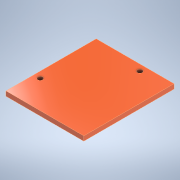
# Autodesk Inventor part: Step-back cover -electronics enc
Saved by Autodesk Inventor 2021 (Build 250183000, 183)
## iProperties
Created: 2020-09-03
Part Number: Step-back cover -electronics enc
Material: Generic
Document SubType Name: Modeling
Designer: jgray
Density: 1 g/cm^3
Appearance: Default
Author: jgray
Autodesk Inventor part; units mm, degrees
ref_plane "YZ Plane" through (0, 0, 0) normal (1, 0, 0) x (0, 1, 0)
ref_plane "XZ Plane" through (0, 0, 0) normal (0, 1, 0) x (-1, 0, 0)
ref_plane "XY Plane" through (0, 0, 0) normal (0, 0, 1) x (1, 0, 0)
sketch "Sketch1" plane through (0, 0, 0) normal (0, 1, 0) x (-1, 0, 0)
  line L0 (0, 0) -> (50, 0)
  line L1 (50, 0) -> (50, -58)
  line L2 (50, -58) -> (0, -58)
  line L3 (0, -58) -> (0, 0)
  line L4 (46, 11.182) -> (46, -76.3332) construction
  line L5 (62.4819, -54) -> (-10.7264, -54) construction
  point P0 (46, -18)
  point P1 (18, -54)
  dimension "d0" = 50
  dimension "d1" = 58
  dimension "d2" = 4
  dimension "d3" = 4
  dimension "d4" = 18
  dimension "d5" = 18
  constraints: 12 end point, 2 horizontal, 2 parallel, 2 point on line, 1 perpendicular, 1 vertical
  measures "d0" distance of L1.end L2.end
  measures "d1" distance of L0.end L1.end
  measures "d2" distance between parallel lines of L1 L4
  measures "d3" distance between parallel lines of L2 L5
  measures "d4" distance from line of L0 point (46, -18)
  measures "d5" distance from line of L3 point (18, -54)
extrude "Extrusion1" add sketch "Sketch1" against normal blind 3
hole "Hole1" at (-46, 0, -18) at (-18, 0, -54) direction (0, -1, 0) diameter 3.2 end through all
body "Solid1"
